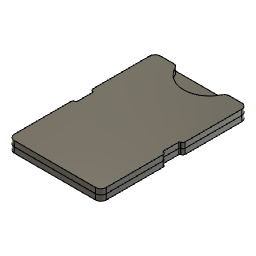
Wallet v1 (Autodesk Fusion 360 design; units mm, degrees)
Autodesk Fusion 360 part; units mm, degrees
note: some values were not read from the file. Set by a fixed rule: which sketch regions a step uses.
sketch "Sketch1" plane through (0, 0, 0) normal (0, 1, 0) x (1, 0, 0)
  line L0 (50.8, -85.725) -> (3.175, -85.725)
  arc A0 (3.175, 0) -> (0, -3.175) centre (3.175, -3.175) ccw
  arc A1 (53.975, -3.175) -> (50.8, 0) centre (50.8, -3.175) ccw
  arc A2 (0, -82.55) -> (3.175, -85.725) centre (3.175, -82.55) ccw
  arc A3 (50.8, -85.725) -> (53.975, -82.55) centre (50.8, -82.55) ccw
  line L1 (3.175, 0) -> (3.81, 0) construction
  line L2 (50.8, 0) -> (27.1399, 0) construction
  line L3 (27.1399, 0) -> (12.8524, 0) construction
  arc A4 (12.8524, 0) -> (41.4274, 0) centre (27.1399, 4.6002) ccw
  line L4 (41.4274, 0) -> (50.8, 0)
  line L5 (12.8524, 0) -> (3.175, 0)
  line L6 (1.27, -37.7825) -> (1.143, -37.7825)
  line L7 (1.778, -38.4175) -> (1.778, -47.3075)
  line L8 (1.143, -47.9425) -> (1.27, -47.9425)
  arc A5 (1.143, -47.9425) -> (1.778, -47.3075) centre (1.143, -47.3075) ccw
  arc A6 (1.778, -38.4175) -> (1.143, -37.7825) centre (1.143, -38.4175) ccw
  line L9 (0, -3.175) -> (0, -36.5125)
  line L10 (0, -49.2125) -> (0, -82.55)
  arc A7 (1.27, -47.9425) -> (0, -49.2125) centre (1.27, -49.2125) ccw
  arc A8 (0, -36.5125) -> (1.27, -37.7825) centre (1.27, -36.5125) ccw
  line L11 (53.975, -82.55) -> (53.975, -49.1998)
  line L12 (52.705, -47.9298) -> (52.832, -47.9298)
  line L13 (52.197, -47.2948) -> (52.197, -38.4048)
  line L14 (52.832, -37.7698) -> (52.705, -37.7698)
  line L15 (53.975, -36.4998) -> (53.975, -3.175)
  arc A9 (53.975, -49.1998) -> (52.705, -47.9298) centre (52.705, -49.1998) ccw
  arc A10 (52.705, -37.7698) -> (53.975, -36.4998) centre (52.705, -36.4998) ccw
  arc A11 (52.197, -47.2948) -> (52.832, -47.9298) centre (52.832, -47.2948) ccw
  arc A12 (52.832, -37.7698) -> (52.197, -38.4048) centre (52.832, -38.4048) ccw
  point P0 (53.975, 0)
  point P1 (0, -85.725)
  point P2 (0, -37.7825)
  point P3 (1.778, -37.7825)
  point P4 (0, -47.9425)
  point P5 (53.975, -47.9298)
  point P6 (52.197, -47.9298)
  point P7 (52.197, -37.7698)
  point P8 (53.975, -37.7698)
  dimension "d1" = 53.975
  dimension "d2" = 85.725
  dimension "d3" = 3.175
  dimension "d4" = 3.175
  dimension "d5" = 3.175
  dimension "d6" = 3.175
  dimension "d8" = 23.6601
  dimension "d9" = 14.2875
  dimension "d13" = 44.7675
  dimension "d14" = 1.778
  dimension "d15" = 10.16
  dimension "d16" = 0.635
  dimension "d17" = 1.27
  dimension "d18" = 1.27
  dimension "d19" = 34.6202
  dimension "d20" = 1.778
  dimension "d21" = 10.16
  dimension "d22" = 1.778
  dimension "d23" = 1.27
  dimension "d24" = 1.27
  dimension "d25" = 0.635
  dimension "d26" = 0.635
  constraint horizontal L0
  constraint coincident P1 L0
  constraint tangent L0 A2
  constraint tangent L0 A3
  constraint tangent A1 L4
  constraint tangent A0 L5
  constraint horizontal L6
  constraint vertical L7
  constraint horizontal L8
  constraint tangent L7 A5
  constraint tangent L8 A5
  constraint coincident P3 L6
  constraint coincident P3 L7
  constraint tangent L6 A6
  constraint tangent L7 A6
  constraint equal A5 A6
  constraint tangent A0 L9
  constraint tangent A2 L10
  constraint coincident P4 L8
  constraint coincident P4 L10
  constraint tangent L8 A7
  constraint tangent L10 A7
  constraint coincident P2 L6
  constraint coincident P2 L9
  constraint tangent L6 A8
  constraint tangent L9 A8
  constraint vertical L11
  constraint perpendicular L11 L12
  constraint perpendicular L12 L13
  constraint perpendicular L13 L14
  constraint tangent A1 L15
  constraint coincident P5 L11
  constraint coincident P5 L12
  constraint tangent L11 A9
  constraint tangent L12 A9
  constraint coincident P8 L14
  constraint coincident P8 L15
  constraint tangent L14 A10
  constraint tangent L15 A10
  constraint coincident P6 L12
  constraint coincident P6 L13
  constraint tangent L12 A11
  constraint tangent L13 A11
  constraint coincident P7 L13
  constraint coincident P7 L14
  constraint tangent L13 A12
  constraint tangent L14 A12
  measures "d1" distance of origin P0
  measures "d2" distance of origin P1
  measures "d3" radius of A0
  measures "d4" radius of A1
  measures "d5" radius of A2
  measures "d6" radius of A3
  measures "d8" distance of A1.end L2.end
  measures "d9" distance of L2.end L3.end
  measures "d13" distance of A2.start P2
  measures "d14" distance of P2 P3
  measures "d15" distance of P2 P4
  measures "d16" radius of A5
  measures "d17" radius of A7
  measures "d18" radius of A8
  measures "d19" distance of A3.end P5
  measures "d20" distance of P5 P6
  measures "d21" distance of P6 P7
  measures "d22" distance of P7 P8
  measures "d23" radius of A9
  measures "d24" radius of A10
  measures "d25" radius of A11
  measures "d26" radius of A12
extrude "Extrude1" add sketch "Sketch1" along normal blind 3.175 makes body 1 in component "Component"
fillet "Fillet1" radius 3.175 2 edges at (41.4274, 1.5875, 0) (12.8524, 1.5875, 0) on bodies 1 in component "Component"
sketch "Sketch2" plane through (0, 0, 0) normal (0, -1, 0) x (1, 0, 0)
  arc A0 (40.7085, 1.8175) -> (43.5787, 0) centre (43.5787, 3.175) ccw
  line L0 (43.5787, 0) -> (50.8, 0)
  arc A1 (50.8, 0) -> (53.975, 3.175) centre (50.8, 3.175) ccw
  arc A2 (53.975, 82.55) -> (50.8, 85.725) centre (50.8, 82.55) ccw
  line L1 (50.8, 85.725) -> (3.175, 85.725)
  arc A3 (3.175, 85.725) -> (0, 82.55) centre (3.175, 82.55) ccw
  arc A4 (0, 3.175) -> (3.175, 0) centre (3.175, 3.175) ccw
  line L2 (3.175, 0) -> (10.7011, 0)
  line L3 (10.7011, 0) -> (44.45, 0)
  line L4 (53.975, 3.175) -> (53.975, 36.4998)
  arc A5 (53.975, 36.4998) -> (52.705, 37.7698) centre (52.705, 36.4998) ccw
  line L5 (52.705, 37.7698) -> (52.832, 37.7698)
  arc A6 (52.197, 38.4048) -> (52.832, 37.7698) centre (52.832, 38.4048) ccw
  line L6 (52.197, 38.4048) -> (52.197, 47.2948)
  arc A7 (52.832, 47.9298) -> (52.197, 47.2948) centre (52.832, 47.2948) ccw
  line L7 (52.832, 47.9298) -> (52.705, 47.9298)
  arc A8 (52.705, 47.9298) -> (53.975, 49.1998) centre (52.705, 49.1998) ccw
  line L8 (53.975, 49.1998) -> (53.975, 82.55)
  line L9 (0, 82.55) -> (0, 49.2125)
  arc A9 (0, 49.2125) -> (1.27, 47.9425) centre (1.27, 49.2125) ccw
  line L10 (1.27, 47.9425) -> (1.143, 47.9425)
  arc A10 (1.778, 47.3075) -> (1.143, 47.9425) centre (1.143, 47.3075) ccw
  line L11 (1.778, 47.3075) -> (1.778, 38.4175)
  arc A11 (1.143, 37.7825) -> (1.778, 38.4175) centre (1.143, 38.4175) ccw
  line L12 (1.143, 37.7825) -> (1.27, 37.7825)
  arc A12 (1.27, 37.7825) -> (0, 36.5125) centre (1.27, 36.5125) ccw
  line L13 (0, 36.5125) -> (0, 3.175)
  constraint coincident L2.end L3.start
  constraint coincident L0 L3.end
  constraint parallel L0 L3
extrude "Extrude1'" add sketch "Sketch2" along normal blind 3.175 separate body makes body 2 in component "Component'"
sketch "Sketch3" plane through (0, -3.175, 0) normal (0, -1, 0) x (1, 0, 0)
  line L0 (1.143, 37.7825) -> (1.27, 37.7825)
  arc A0 (1.27, 37.7825) -> (0, 36.5125) centre (1.27, 36.5125) ccw
  line L1 (0, 36.5125) -> (0, 3.175)
  arc A1 (0, 3.175) -> (3.175, 0) centre (3.175, 3.175) ccw
  line L2 (3.175, 0) -> (50.8, 0)
  arc A2 (50.8, 0) -> (53.975, 3.175) centre (50.8, 3.175) ccw
  line L3 (53.975, 3.175) -> (53.975, 36.4998)
  arc A3 (53.975, 36.4998) -> (52.705, 37.7698) centre (52.705, 36.4998) ccw
  line L4 (52.705, 37.7698) -> (52.832, 37.7698)
  arc A4 (52.197, 38.4048) -> (52.832, 37.7698) centre (52.832, 38.4048) ccw
  line L5 (52.197, 38.4048) -> (52.197, 47.2948)
  arc A5 (52.832, 47.9298) -> (52.197, 47.2948) centre (52.832, 47.2948) ccw
  line L6 (52.832, 47.9298) -> (52.705, 47.9298)
  arc A6 (52.705, 47.9298) -> (53.975, 49.1998) centre (52.705, 49.1998) ccw
  line L7 (53.975, 49.1998) -> (53.975, 82.55)
  arc A7 (53.975, 82.55) -> (50.8, 85.725) centre (50.8, 82.55) ccw
  line L8 (50.8, 85.725) -> (3.175, 85.725)
  arc A8 (3.175, 85.725) -> (0, 82.55) centre (3.175, 82.55) ccw
  line L9 (0, 82.55) -> (0, 49.2125)
  arc A9 (0, 49.2125) -> (1.27, 47.9425) centre (1.27, 49.2125) ccw
  line L10 (1.27, 47.9425) -> (1.143, 47.9425)
  arc A10 (1.778, 47.3075) -> (1.143, 47.9425) centre (1.143, 47.3075) ccw
  line L11 (1.778, 47.3075) -> (1.778, 38.4175)
  arc A11 (1.143, 37.7825) -> (1.778, 38.4175) centre (1.143, 38.4175) ccw
sketch "Sketch4" plane through (0, 3.175, 0) normal (0, 1, 0) x (-1, 0, 0)
  arc A0 (-13.5713, 1.8175) -> (-10.7011, 0) centre (-10.7011, 3.175) ccw
  line L0 (-10.7011, 0) -> (-3.175, 0)
  arc A1 (-3.175, 0) -> (0, 3.175) centre (-3.175, 3.175) ccw
  line L1 (0, 3.175) -> (0, 36.5125)
  arc A2 (0, 36.5125) -> (-1.27, 37.7825) centre (-1.27, 36.5125) ccw
  line L2 (-1.27, 37.7825) -> (-1.143, 37.7825)
  arc A3 (-1.778, 38.4175) -> (-1.143, 37.7825) centre (-1.143, 38.4175) ccw
  line L3 (-1.778, 38.4175) -> (-1.778, 47.3075)
  arc A4 (-1.143, 47.9425) -> (-1.778, 47.3075) centre (-1.143, 47.3075) ccw
  line L4 (-1.143, 47.9425) -> (-1.27, 47.9425)
  arc A5 (-1.27, 47.9425) -> (0, 49.2125) centre (-1.27, 49.2125) ccw
  line L5 (0, 49.2125) -> (0, 82.55)
  arc A6 (0, 82.55) -> (-3.175, 85.725) centre (-3.175, 82.55) ccw
  line L6 (-3.175, 85.725) -> (-50.8, 85.725)
  arc A7 (-50.8, 85.725) -> (-53.975, 82.55) centre (-50.8, 82.55) ccw
  line L7 (-53.975, 82.55) -> (-53.975, 49.1998)
  arc A8 (-53.975, 49.1998) -> (-52.705, 47.9298) centre (-52.705, 49.1998) ccw
  line L8 (-52.705, 47.9298) -> (-52.832, 47.9298)
  arc A9 (-52.197, 47.2948) -> (-52.832, 47.9298) centre (-52.832, 47.2948) ccw
  line L9 (-52.197, 47.2948) -> (-52.197, 38.4048)
  arc A10 (-52.832, 37.7698) -> (-52.197, 38.4048) centre (-52.832, 38.4048) ccw
  line L10 (-52.832, 37.7698) -> (-52.705, 37.7698)
  arc A11 (-52.705, 37.7698) -> (-53.975, 36.4998) centre (-52.705, 36.4998) ccw
  line L11 (-53.975, 36.4998) -> (-53.975, 3.175)
  arc A12 (-53.975, 3.175) -> (-50.8, 0) centre (-50.8, 3.175) ccw
  line L12 (-50.8, 0) -> (-43.5787, 0)
  arc A13 (-43.5787, 0) -> (-40.7085, 1.8175) centre (-43.5787, 3.175) ccw
  arc A14 (-13.5713, 1.8175) -> (-40.7085, 1.8175) centre (-27.1399, -4.6002) ccw
component "Component" placed x (1, 0, 0) y (0, 1, 0) z (0, 0, 1) at (0, 0, 0)
component "Component'" placed x (1, 0, 0) y (0, 1, 0) z (0, 0, 1) at (0, 0, 0)
equation "d8 = ( 1.863 / 2 ) * 1 in"
equation "d9 = ( 1.125 / 2 ) * 1 in"
equation "d13 = ( 3.125 / 2 ) * 1 in + 0.2 in"
equation "d19 = 1.763 in - 0.4 in"
